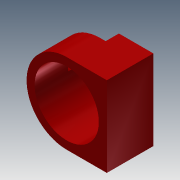
# Autodesk Inventor part: HbThumbMetacarpalPhalanxCover01
Saved by Autodesk Inventor 2015 SP1 (Build 190203100, 203)
## iProperties
Created: 2015-09-12
Part Number: HbThumbMetacarpalPhalanxCover01
Material: ABS プラスチック
Document SubType Name: Modeling
Designer: Yamaura
Density: 1.06 g/cm^3
Appearance: 滑らか - 赤
Author: Yamaura
Autodesk Inventor part; units mm, degrees
ref_plane "YZ Plane" through (0, 0, 0) normal (1, 0, 0) x (0, 1, 0)
ref_plane "XZ Plane" through (0, 0, 0) normal (0, 1, 0) x (-1, 0, 0)
ref_plane "XY Plane" through (0, 0, 0) normal (0, 0, 1) x (1, 0, 0)
sketch "スケッチ1" plane through (0, 0, 0) normal (0, 0, 1) x (1, 0, 0)
  circle A0 centre (0, 0) radius 8
  line L0 (-10, 10) -> (10, 10)
  line L1 (10, 10) -> (10, -10)
  line L2 (10, -10) -> (-10, -10)
  line L3 (-10, -10) -> (-10, 10)
  dimension "d0" = 16
  dimension "d1" = 10
  dimension "d2" = 10
  dimension "d3" = 20
  dimension "d4" = 10
  constraints: 8 end point, 2 parallel, 1 centre point, 1 coincident, 1 horizontal, 1 perpendicular
  measures "d0" diameter of A0
  measures "d1" distance from line of L3 point (0, 0)
  measures "d2" distance from line of L0 point (0, 0)
  measures "d3" distance of L2.end L0.start
  measures "d4" distance from line of L1 point (0, 0)
extrude "押し出し1" add sketch "スケッチ1" along normal blind 2
sketch "スケッチ2" plane through (0, 0, 0) normal (0, 0, 1) x (1, 0, 0)
  circle A0 centre (0, 0) radius 8
  circle A1 centre (0, 0) radius 10
  line L0 (10, 10) -> (-10, 10) projected
  line L1 (0, 10) -> (0, 10)
  line L2 (0, -10) -> (0, -10)
  line L3 (0, 10) -> (0, 8)
  circle A2 centre (0, 0) radius 8 projected
  line L4 (-10, 10) -> (10, 10) projected
  line L5 (10, 10) -> (10, -10) projected
  line L6 (10, -10) -> (-10, -10) projected
  line L7 (-10, -10) -> (-10, 10) projected
  line L8 (0, -10) -> (10, -10)
  line L9 (10, -10) -> (10, 10)
  line L10 (-10, -10) -> (10, -10) projected
  line L11 (10, 10) -> (0, 10)
  dimension "d7" = 16
  dimension "d8" = 20
  dimension "d29" = 0
  constraints: 12 end point, 4 perpendicular, 2 coincident, 2 midpoint, 2 point on circle, 1 centre point, 1 horizontal, 1 vertical alignment, 2 other
  measures "d8" diameter of A1
  measures "d29" distance of L1.start L1.end
extrude "押し出し2" add sketch "スケッチ2" against normal blind 9.6 contours A1 | L5 L6 A1 | A1 L0 L5
delete faces "削除1" heal yes whole lump no faces at (-8.0177, 8.0177, 0) (-8.0177, -8.0177, 0)
sketch "スケッチ4" plane through (0, 0, -9.6) normal (0, 0, -1) x (0, 1, 0)
  line L0 (0, 0) -> (9.0631, -4.2262)
  line L1 (0, 0) -> (10, 0) construction
  line L2 (11.896, -9.9819) -> (15.919, -1.3546)
  line L3 (15.919, -1.3546) -> (2.3244, 4.9847)
  line L4 (2.3244, 4.9847) -> (0, 0)
  line L5 (0, 0) -> (5.7358, -8.1915)
  line L6 (0, 0) -> (10, 0) construction
  line L7 (0, 0) -> (-4.5053, -3.1547)
  line L8 (-4.5053, -3.1547) -> (4.0983, -15.442)
  line L9 (11.896, -9.9819) -> (4.0983, -15.442)
  dimension "d17" = 10
  dimension "d20" = 5.5
  dimension "d24" = 15
  dimension "d25" = 10
  dimension "d27" = 5.5
  dimension "d28" = 15
  dimension "d30" = 30
  dimension "d31" = 25
  constraints: 20 end point, 3 parallel, 3 perpendicular, 2 equal length, 2 horizontal, 2 point on line
  measures "d17" distance of L0.start L0.end
  measures "d20" distance between parallel lines of L3 L0
  measures "d24" distance of L2.end L3.end
  measures "d25" distance of L4.end L5.end
  measures "d27" distance of L4.end L7.end
  measures "d28" distance of L7.end L8.end
  measures "d30" angle of L5 L0
  measures "d31" angle of L0 L1
extrude "押し出し4" cut sketch "スケッチ4" against normal blind 3.3
